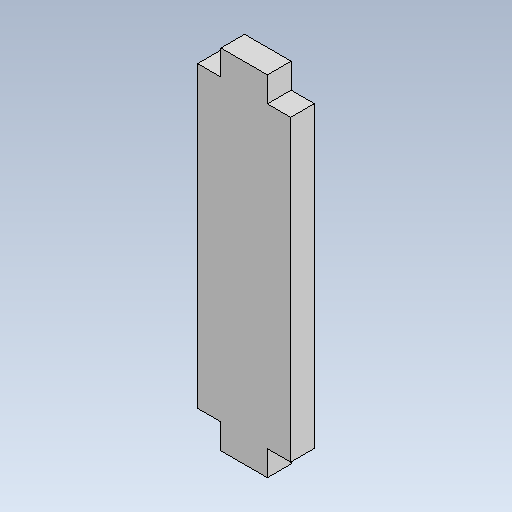
# Autodesk Inventor part: custom standoffs
Saved by Autodesk Inventor 2025 (Build 290162000, 162)
## iProperties
Created: 2024-08-13
Part Number: custom standoffs
Material: Polycarbonate, Smoke
Document SubType Name: Modeling
Designer: PC
Density: 1.2 g/cm^3
Appearance: Default
Author: PC
Autodesk Inventor part; units mm, degrees
ref_plane "YZ Plane" through (0, 0, 0) normal (1, 0, 0) x (0, 1, 0)
ref_plane "XZ Plane" through (0, 0, 0) normal (0, 1, 0) x (-1, 0, 0)
ref_plane "XY Plane" through (0, 0, 0) normal (0, 0, 1) x (1, 0, 0)
sketch "Sketch1" plane through (0, 0, 0) normal (0, 0, 1) x (1, 0, 0)
  line L0 (-5, 0) -> (-15, 0)
  line L1 (0, 69.6) -> (0, 5.4)
  line L2 (-20, 69.6) -> (-15, 69.6)
  line L3 (-15, 69.6) -> (-15, 75)
  line L4 (-15, 75) -> (-5, 75)
  line L5 (-5, 75) -> (-5, 69.6)
  line L6 (-5, 69.6) -> (0, 69.6)
  line L7 (-20, 69.6) -> (-20, 5.4)
  line L8 (-33.5059, 37.5) -> (28.6697, 37.5) construction
  line L9 (0, 5.4) -> (0, 69.6)
  line L10 (-20, 5.4) -> (-15, 5.4)
  line L11 (-15, 5.4) -> (-15, 0)
  line L12 (-15, 0) -> (-5, 0)
  line L13 (-5, 0) -> (-5, 5.4)
  line L14 (-5, 5.4) -> (0, 5.4)
  line L15 (-20, 5.4) -> (-20, 69.6)
  point P0 (0, 0)
  dimension "d3" = 10
  dimension "d4" = 75
  dimension "d5" = 5.4
  dimension "d6" = 37.5
  dimension "d7" = 20
  dimension "d8" = 20
  dimension "d9" = 5
  constraints: 32 end point, 6 symmetric about line, 4 point on line, 3 horizontal, 3 perpendicular, 1 vertical
  measures "d3" distance of L3.end L4.end
  measures "d4" vertical distance of point (0, 0) L4.end
  measures "d5" distance of L2.end L3.end
  measures "d6" distance from line of point (0, 0) L8
  measures "d7" distance from line of point (0, 0) L15
  measures "d8" distance between parallel lines of L7 L1
  measures "d9" distance between parallel lines of L5 L1
extrude "Extrusion1" add sketch "Sketch1" along normal blind 5.1
body "Solid1"
